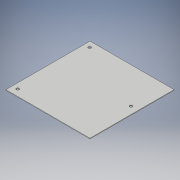
# Autodesk Inventor part: 4xSplitter
Saved by Autodesk Inventor 2018 (Build 220112000, 112)
## iProperties
Created: 2018-04-06
Part Number: 4xSplitter
Material: Generic
Document SubType Name: Modeling
Designer: bbramman
Density: 1 g/cm^3
Appearance: Default
Author: bbramman
Autodesk Inventor part; units mm, degrees
ref_plane "YZ Plane" through (0, 0, 0) normal (1, 0, 0) x (0, 1, 0)
ref_plane "XZ Plane" through (0, 0, 0) normal (0, 1, 0) x (-1, 0, 0)
ref_plane "XY Plane" through (0, 0, 0) normal (0, 0, 1) x (1, 0, 0)
sketch "Sketch2" plane through (0, 0, 0) normal (0, 1, 0) x (-1, 0, 0)
  line L0 (-50, 50) -> (50, 50)
  line L1 (50, 50) -> (50, -50)
  line L2 (50, -50) -> (-50, -50)
  line L3 (-50, -50) -> (-50, 50)
  line L4 (-50, 50) -> (50, -50) construction
  line L5 (50, 50) -> (-50, -50) construction
  point P0 (0, 0)
  dimension "d4" = 100
  dimension "d5" = 100
  constraints: 12 end point, 2 midpoint, 2 parallel, 1 horizontal, 1 perpendicular
  measures "d4" distance of L1.end L2.end
  measures "d5" distance of L0.end L1.end
extrude "Extrusion2" add sketch "Sketch2" along normal mid plane 0.7874
sketch "Sketch3" plane through (0, 0.3937, 0) normal (0, 1, 0) x (1, 0, 0)
  circle A0 centre (41.4401, 7.4041) radius 1.6319
  circle A1 centre (-43.6499, -42.3799) radius 1.632
  circle A2 centre (-43.6499, 43.2181) radius 1.632
  point P0 (0, 0)
  dimension "d8" = 3.2639
  dimension "d9" = 3.2639
  dimension "d10" = 3.2639
  constraints: 3 centre point
  measures "d8" diameter of A0
  measures "d9" diameter of A1
  measures "d10" diameter of A2
extrude "Extrusion3" cut sketch "Sketch3" against normal through all
body "Solid2"
